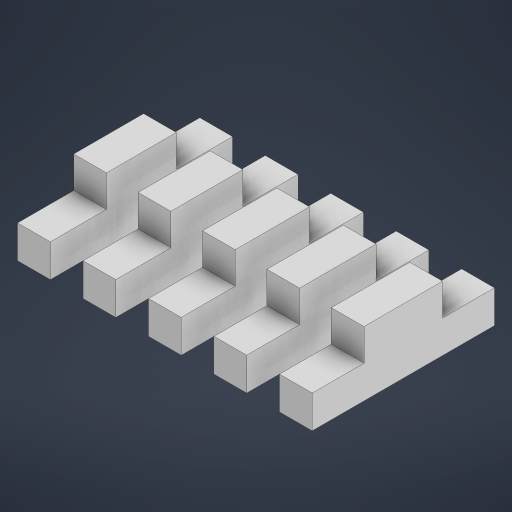
# Autodesk Inventor part: press_fit_test_2
Saved by Autodesk Inventor 2023 (Build 270158000, 158)
## iProperties
Created: 2022-05-10
Part Number: press_fit_test_2
Material: Generic
Document SubType Name: Modeling
Designer: Haroon Nawaz
Density: 1 g/cm^3
Appearance: Default
Author: Haroon Nawaz
Autodesk Inventor part; units mm, degrees
ref_plane "YZ Plane" through (0, 0, 0) normal (1, 0, 0) x (0, 1, 0)
ref_plane "XZ Plane" through (0, 0, 0) normal (0, 1, 0) x (-1, 0, 0)
ref_plane "XY Plane" through (0, 0, 0) normal (0, 0, 1) x (1, 0, 0)
ref_plane "Work Plane2" through (-3.5, 0, -12.7) normal (-1, 0, 0) x (0, 0, 1)
sketch "Sketch7" plane through (-3.5, 0, -12.7) normal (-1, 0, 0) x (0, 0, 1)
  line L0 (4.35, 1.5) -> (8.35, 1.5) projected
  line L1 (8.35, 3) -> (8.35, 2.95)
  line L2 (4.35, 2.95) -> (4.35, 3)
  line L3 (0, 0) -> (0, 3) projected
  line L4 (4.35, 3) -> (4.35, 1.5) projected
  line L5 (0, 1.5) -> (4.35, 1.5)
  line L6 (4.55, 1.5) -> (8.15, 1.5)
  line L7 (8.35, 1.5) -> (12.7, 1.5)
  line L8 (12.7, 3) -> (12.7, 0) projected
  line L9 (4.35, 1.5) -> (0, 1.5)
  line L10 (12.7, 0) -> (0, 0) projected
  line L11 (2.175, 1.5) -> (8.15, 1.5)
  line L12 (10.525, 1.5) -> (10.525, 0)
  line L13 (10.525, 0) -> (2.175, 0)
  line L14 (2.175, 0) -> (2.175, 1.5)
  line L15 (4.35, 1.5) -> (4.55, 1.5)
  line L16 (4.55, 1.5) -> (4.55, 3)
  line L17 (8.35, 1.5) -> (8.15, 1.5)
  line L18 (8.15, 1.5) -> (8.15, 2.95)
  line L19 (4.55, 3) -> (4.55, 2.95)
  line L20 (4.55, 2.95) -> (8.15, 2.95)
  line L21 (8.35, 1.5) -> (8.15, 1.5)
  line L22 (4.55, 1.5) -> (4.35, 1.5)
  point P0 (4.55, 1.5)
  dimension "d66" = 0.2
  dimension "d67" = 0.2
  dimension "d68" = 0.05
  constraints: 36 end point, 5 point on line, 4 midpoint, 3 parallel, 3 perpendicular, 2 collinear, 2 horizontal
  measures "d66" distance of L6.start L9.start
  measures "d67" distance of L6.end L0.end
  measures "d68" distance of L16.end L19.end
extrude "Extrusion6" add sketch "Sketch7" along normal blind 1.5 contours L0 L7 L12 L10 L14 L5 | L16 L20 L18 L0
ref_plane "Work Plane3" through (-7, 0, -12.7) normal (-1, 0, 0) x (0, 0, 1)
pattern_linear "Rectangular Pattern2" count 5 spacing 3 along (-1, 0, 0) of "Extrusion6"
thicken "Thicken10" operation cut thickness 0.05 both sides no extend neighbours no toward (0, 0, 1) faces at (-7, 2.4667, -8.15)
thicken "Thicken11" operation cut thickness 0.1 both sides no extend neighbours no toward (0, 0, 1) faces at (-10, 2.4667, -8.15)
thicken "Thicken12" operation cut thickness 0.15 both sides no extend neighbours no toward (0, 0, 1) faces at (-13, 2.4667, -8.15)
thicken "Thicken13" operation cut thickness 0.2 both sides no extend neighbours no toward (0, 0, 1) faces at (-16, 2.4667, -8.15)
thicken "Thicken14" operation cut thickness 0.2 both sides no extend neighbours no toward (0, 0, -1) faces at (-16, 1.9833, -4.55)
thicken "Thicken15" operation cut thickness 0.15 both sides no extend neighbours no toward (0, 0, -1) faces at (-13, 1.9833, -4.55)
thicken "Thicken16" operation cut thickness 0.1 both sides no extend neighbours no toward (0, 0, -1) faces at (-10, 1.9833, -4.55)
thicken "Thicken17" operation cut thickness 0.05 both sides no extend neighbours no toward (0, 0, -1) faces at (-7, 1.9833, -4.55)
sketch "Sketch14" plane through (-3.5, 0, -10.525) normal (0, -1, 0) x (1, 0, 0)
  line L0 (-1.1, 7.8212) -> (-0.4, 7.8212)
  line L1 (-0.4, 7.8212) -> (-0.4, 7.2079)
  line L2 (-0.4, 7.2079) -> (-1.1, 7.2079)
  line L3 (-1.1, 7.2079) -> (-1.1, 7.8212)
  line L4 (-1.5, 0) -> (-1.5, 8.35) projected
  line L5 (0, 0) -> (0, 8.35) projected
  line L6 (-4.1, 7.8212) -> (-3.4, 7.8212)
  line L7 (-3.4, 7.8212) -> (-3.4, 7.2079)
  line L8 (-3.4, 7.2079) -> (-4.1, 7.2079)
  line L9 (-4.1, 7.2079) -> (-4.1, 7.8212)
  line L10 (-7.1, 7.8212) -> (-6.4, 7.8212)
  line L11 (-6.4, 7.8212) -> (-6.4, 7.2079)
  line L12 (-6.4, 7.2079) -> (-7.1, 7.2079)
  line L13 (-7.1, 7.2079) -> (-7.1, 7.8212)
  line L14 (-10.1, 7.8212) -> (-9.4, 7.8212)
  line L15 (-9.4, 7.8212) -> (-9.4, 7.2079)
  line L16 (-9.4, 7.2079) -> (-10.1, 7.2079)
  line L17 (-10.1, 7.2079) -> (-10.1, 7.8212)
  line L18 (-13.1, 7.8212) -> (-12.4, 7.8212)
  line L19 (-12.4, 7.8212) -> (-12.4, 7.2079)
  line L20 (-12.4, 7.2079) -> (-13.1, 7.2079)
  line L21 (-13.1, 7.2079) -> (-13.1, 7.8212)
  line L22 (-4.1, 6.3212) -> (-3.4, 6.3212)
  line L23 (-4.1, 5.7079) -> (-4.1, 6.3212)
  line L24 (-3.4, 5.7079) -> (-4.1, 5.7079)
  line L25 (-3.4, 6.3212) -> (-3.4, 5.7079)
  line L26 (-6.4, 6.3212) -> (-6.4, 5.7079)
  line L27 (-7.1, 5.7079) -> (-7.1, 6.3212)
  line L28 (-7.1, 6.3212) -> (-6.4, 6.3212)
  line L29 (-6.4, 5.7079) -> (-7.1, 5.7079)
  line L30 (-6.4, 4.8212) -> (-6.4, 4.2079)
  line L31 (-7.1, 4.2079) -> (-7.1, 4.8212)
  line L32 (-7.1, 4.8212) -> (-6.4, 4.8212)
  line L33 (-6.4, 4.2079) -> (-7.1, 4.2079)
  line L34 (-10.1, 6.3212) -> (-9.4, 6.3212)
  line L35 (-9.4, 6.3212) -> (-9.4, 5.7079)
  line L36 (-9.4, 5.7079) -> (-10.1, 5.7079)
  line L37 (-10.1, 5.7079) -> (-10.1, 6.3212)
  line L38 (-10.1, 4.8212) -> (-9.4, 4.8212)
  line L39 (-9.4, 4.8212) -> (-9.4, 4.2079)
  line L40 (-9.4, 4.2079) -> (-10.1, 4.2079)
  line L41 (-10.1, 4.2079) -> (-10.1, 4.8212)
  line L42 (-10.1, 3.3212) -> (-9.4, 3.3212)
  line L43 (-9.4, 3.3212) -> (-9.4, 2.7079)
  line L44 (-9.4, 2.7079) -> (-10.1, 2.7079)
  line L45 (-10.1, 2.7079) -> (-10.1, 3.3212)
  line L46 (-12.4, 5.7079) -> (-13.1, 5.7079)
  line L47 (-12.4, 6.3212) -> (-12.4, 5.7079)
  line L48 (-13.1, 5.7079) -> (-13.1, 6.3212)
  line L49 (-13.1, 6.3212) -> (-12.4, 6.3212)
  line L50 (-12.4, 4.2079) -> (-13.1, 4.2079)
  line L51 (-12.4, 4.8212) -> (-12.4, 4.2079)
  line L52 (-13.1, 4.2079) -> (-13.1, 4.8212)
  line L53 (-13.1, 4.8212) -> (-12.4, 4.8212)
  line L54 (-12.4, 2.7079) -> (-13.1, 2.7079)
  line L55 (-12.4, 3.3212) -> (-12.4, 2.7079)
  line L56 (-13.1, 2.7079) -> (-13.1, 3.3212)
  line L57 (-13.1, 3.3212) -> (-12.4, 3.3212)
  line L58 (-12.4, 1.2079) -> (-13.1, 1.2079)
  line L59 (-12.4, 1.8212) -> (-12.4, 1.2079)
  line L60 (-13.1, 1.2079) -> (-13.1, 1.8212)
  line L61 (-13.1, 1.8212) -> (-12.4, 1.8212)
  point P0 (3.5, 10.525)
  dimension "d88" = 0.4
  dimension "d89" = 0.4
  dimension "d92" = 3
  dimension "d99" = 1.5
  dimension "d106" = 1.5
  dimension "d113" = 1.5
  dimension "d120" = 1.5
  constraints: 120 end point, 5 collinear, 4 vertical, 2 horizontal, 2 parallel, 1 perpendicular, 107 other
  measures "d88" distance between parallel lines of L4 L3
  measures "d89" distance between parallel lines of L5 L1
  measures "d92" distance of L0.start L6.start
  measures "d99" distance of L7.end L24.start
  measures "d106" distance of L11.end L26.end
  measures "d113" distance of L14.start L34.start
  measures "d120" distance of L19.end L46.start
extrude "Extrusion10" cut sketch "Sketch14" against normal blind 1
body "Solid1"
